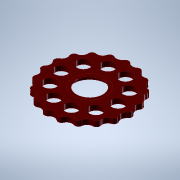
# Autodesk Inventor part: Rotor
Saved by Autodesk Inventor 2021 (Build 250183000, 183)
## iProperties
Created: 2022-08-28
Part Number: Rotor
Material: Ogólny
Document SubType Name: Modeling
Designer: MicnedSQ
Density: 1 g/cm^3
Appearance: Jasnoczerwona
Author: MicnedSQ
## iProperties of the stored document _Drukowanie 3D.ipt
Created: 2022-08-31
Part Number: _Drukowanie 3D
Material: Ogólny
Document SubType Name: Modeling
Designer: MicnedSQ
Density: 1 g/cm^3
Appearance: Domyślna
Author: MicnedSQ
Autodesk Inventor part; units mm, degrees
ref_plane "YZ Plane" through (0, 0, 0) normal (1, 0, 0) x (0, 1, 0)
ref_plane "XZ Plane" through (0, 0, 0) normal (0, 1, 0) x (-1, 0, 0)
ref_plane "XY Plane" through (0, 0, 0) normal (0, 0, 1) x (1, 0, 0)
sketch "Szkic1" plane through (0, 0, 0) normal (0, 1, 0) x (-1, 0, 0)
  spline S0 degree 5 poles (38.5, 0) (38.486, -0.9355) (38.7301, -1.8055) (39.0456, -2.7484) (39.8212, -3.5737) (40.5099, -4.4698) (40.6142, -4.6562) (40.8333, -5.1108) (40.9496, -5.6078) (40.9887, -5.8989) (41.0044, -6.5159) (40.8948, -7.12) (40.8044, -7.4298) (40.5885, -7.9454) (40.2744, -8.4095) (40.1203, -8.5919) (39.6992, -9.0108) (39.1783, -9.3014) (38.8791, -9.4777) (37.3997, -10.474) (36.3142, -11.9401) (35.8618, -13.4696) (36.0404, -15.1944) (36.6496, -16.773) (36.7512, -17.0218) (36.9128, -17.5238) (36.9474, -18.0505) (36.941, -18.3049) (36.8653, -18.8806) (36.6769, -19.4279) (36.5371, -19.7236) (36.2216, -20.2389) (35.8062, -20.6826) (35.5946, -20.8646) (35.1852, -21.1554) (34.728, -21.3438) (34.5206, -21.4137) (33.1558, -21.698) (31.793, -22.0921) (30.8042, -22.9138) (29.6475, -24.3964) (29.2399, -26.2198) (29.1454, -26.8625) (29.2627, -27.7313) (29.2011, -28.5914) (29.1537, -28.807) (29.0102, -29.3081) (28.7594, -29.7733) (28.5887, -30.0266) (28.1871, -30.5007) (27.6995, -30.8822) (27.4328, -31.0484) (26.9472, -31.2834) (26.426, -31.4138) (26.2028, -31.4498) (25.4759, -31.4825) (24.7564, -31.3259) (24.2597, -31.3096) (22.4191, -31.3724) (20.7296, -32.1668) (19.635, -33.1235) (18.9622, -34.5428) (18.5386, -36.0225) (18.4616, -36.2397) (18.2536, -36.6941) (17.9463, -37.0929) (17.7617, -37.2901) (17.31, -37.6816) (16.7902, -37.973) (16.4887, -38.1014) (15.923, -38.2724) (15.3331, -38.3261) (15.0679, -38.3226) (14.5636, -38.2676) (14.0874, -38.0997) (13.8701, -37.9997) (12.443, -37.2851) (10.8679, -36.8588) (9.3686, -37.0732) (7.6938, -37.8748) (6.4646, -39.2255) (6.191, -39.5691) (5.8381, -40.1537) (5.3451, -40.617) (5.1626, -40.7567) (4.6999, -41.0453) (4.1885, -41.2353) (3.8803, -41.3129) (3.269, -41.3994) (2.6488, -41.3603) (2.3525, -41.3079) (1.8482, -41.1691) (1.3948, -40.9271) (1.2077, -40.8149) (0.4846, -40.2055) (-0.1383, -39.4759) (-0.7752, -39.0861) (-2.4573, -38.2565) (-4.3399, -38.2442) (-5.5025, -38.4561) (-6.6123, -39.1858) (-7.6837, -39.9373) (-7.877, -40.0356) (-8.3311, -40.2356) (-8.8273, -40.3293) (-9.1094, -40.3566) (-9.7214, -40.3481) (-10.3147, -40.2173) (-10.6241, -40.1134) (-11.1431, -39.8723) (-11.6056, -39.5317) (-11.7893, -39.3635) (-12.1573, -38.9616) (-12.4116, -38.4794) (-12.5331, -38.216) (-13.3167, -36.6788) (-14.5397, -35.4012) (-16.0003, -34.7345) (-17.7967, -34.6208) (-19.4972, -35.064) (-19.7997, -35.1602) (-20.3453, -35.323) (-20.9136, -35.3357) (-21.1567, -35.3204) (-21.7162, -35.2238) (-22.2434, -35.0197) (-22.5316, -34.8691) (-23.0397, -34.5308) (-23.4728, -34.093) (-23.6512, -33.8673) (-23.9293, -33.4414) (-24.1006, -32.9737) (-24.1648, -32.7676) (-24.3431, -31.5633) (-24.4967, -30.3342) (-25.0291, -29.4057) (-26.199, -27.9263) (-27.907, -27.1334) (-28.7075, -26.8539) (-29.7585, -26.8736) (-30.7855, -26.7673) (-30.995, -26.7101) (-31.4778, -26.5536) (-31.9228, -26.2883) (-32.1623, -26.1137) (-32.6199, -25.6947) (-32.9801, -25.1958) (-33.1397, -24.9172) (-33.3591, -24.4108) (-33.4741, -23.8696) (-33.499, -23.6372) (-33.5086, -23.0043) (-33.3431, -22.3895) (-33.2706, -22.0056) (-33.0507, -20.2136) (-33.4922, -18.4251) (-34.3338, -17.1132) (-35.7229, -16.1585) (-37.2593, -15.5672) (-37.4951, -15.4755) (-37.9565, -15.2464) (-38.3521, -14.9145) (-38.5347, -14.7296) (-38.9012, -14.2715) (-39.1677, -13.7506) (-39.2841, -13.4443) (-39.4357, -12.8633) (-39.467, -12.2611) (-39.4522, -11.9868) (-39.3778, -11.4905) (-39.1962, -11.0287) (-39.0981, -10.8276) (-38.3366, -9.572) (-37.7222, -8.2083) (-37.7055, -6.8353) (-38.1425, -5.013) (-39.2807, -3.5467) (-39.6615, -3.1219) (-40.322, -2.6634) (-40.8495, -2.0714) (-40.9748, -1.8868) (-41.2394, -1.4286) (-41.4036, -0.9206) (-41.4684, -0.6174) (-41.5316, 0) (-41.4684, 0.6174) (-41.4036, 0.9206) (-41.2394, 1.4286) (-40.9748, 1.8868) (-40.8495, 2.0714) (-40.322, 2.6634) (-39.6615, 3.1219) (-39.2807, 3.5467) (-38.1425, 5.013) (-37.7055, 6.8353) (-37.7222, 8.2083) (-38.3366, 9.572) (-39.0981, 10.8276) (-39.1962, 11.0287) (-39.3778, 11.4905) (-39.4522, 11.9868) (-39.467, 12.2611) (-39.4357, 12.8633) (-39.2841, 13.4443) (-39.1677, 13.7506) (-38.9012, 14.2715) (-38.5347, 14.7296) (-38.3521, 14.9145) (-37.9565, 15.2464) (-37.4951, 15.4755) (-37.2593, 15.5672) (-35.7229, 16.1585) (-34.3338, 17.1132) (-33.4922, 18.4251) (-33.0507, 20.2136) (-33.2706, 22.0056) (-33.3431, 22.3895) (-33.5086, 23.0043) (-33.499, 23.6372) (-33.4741, 23.8696) (-33.3591, 24.4108) (-33.1397, 24.9172) (-32.9801, 25.1958) (-32.6199, 25.6947) (-32.1623, 26.1137) (-31.9228, 26.2883) (-31.4778, 26.5536) (-30.995, 26.7101) (-30.7855, 26.7673) (-29.7585, 26.8736) (-28.7075, 26.8539) (-27.907, 27.1334) (-26.199, 27.9263) (-25.0291, 29.4057) (-24.4967, 30.3342) (-24.3431, 31.5633) (-24.1648, 32.7676) (-24.1006, 32.9737) (-23.9293, 33.4414) (-23.6512, 33.8673) (-23.4728, 34.093) (-23.0397, 34.5308) (-22.5316, 34.8691) (-22.2434, 35.0197) (-21.7162, 35.2238) (-21.1567, 35.3204) (-20.9136, 35.3357) (-20.3453, 35.323) (-19.7997, 35.1602) (-19.4972, 35.064) (-17.7967, 34.6208) (-16.0003, 34.7345) (-14.5397, 35.4012) (-13.3167, 36.6788) (-12.5331, 38.216) (-12.4116, 38.4794) (-12.1573, 38.9616) (-11.7893, 39.3635) (-11.6056, 39.5317) (-11.1431, 39.8723) (-10.6241, 40.1134) (-10.3147, 40.2173) (-9.7214, 40.3481) (-9.1094, 40.3566) (-8.8273, 40.3293) (-8.3311, 40.2356) (-7.877, 40.0356) (-7.6837, 39.9373) (-6.6123, 39.1858) (-5.5025, 38.4561) (-4.3399, 38.2442) (-2.4573, 38.2565) (-0.7752, 39.0861) (-0.1383, 39.4759) (0.4846, 40.2055) (1.2077, 40.8149) (1.3948, 40.9271) (1.8482, 41.1691) (2.3525, 41.3079) (2.6488, 41.3603) (3.269, 41.3994) (3.8803, 41.3129) (4.1885, 41.2353) (4.6999, 41.0453) (5.1626, 40.7567) (5.3451, 40.617) (5.8381, 40.1537) (6.191, 39.5691) (6.4646, 39.2255) (7.6938, 37.8748) (9.3686, 37.0732) (10.8679, 36.8588) (12.443, 37.2851) (13.8701, 37.9997) (14.0874, 38.0997) (14.5636, 38.2676) (15.0679, 38.3226) (15.3331, 38.3261) (15.923, 38.2724) (16.4887, 38.1014) (16.7902, 37.973) (17.31, 37.6816) (17.7617, 37.2901) (17.9463, 37.0929) (18.2536, 36.6941) (18.4616, 36.2397) (18.5386, 36.0225) (18.9622, 34.5428) (19.635, 33.1235) (20.7296, 32.1668) (22.4191, 31.3724) (24.2597, 31.3096) (24.7564, 31.3259) (25.4759, 31.4825) (26.2028, 31.4498) (26.426, 31.4138) (26.9472, 31.2834) (27.4328, 31.0484) (27.6995, 30.8822) (28.1871, 30.5007) (28.5887, 30.0266) (28.7594, 29.7733) (29.0102, 29.3081) (29.1537, 28.807) (29.2011, 28.5914) (29.2627, 27.7313) (29.1454, 26.8625) (29.2399, 26.2198) (29.6475, 24.3964) (30.8042, 22.9138) (31.793, 22.0921) (33.1558, 21.698) (34.5206, 21.4137) (34.728, 21.3438) (35.1852, 21.1554) (35.5946, 20.8646) (35.8062, 20.6826) (36.2216, 20.2389) (36.5371, 19.7236) (36.6769, 19.4279) (36.8653, 18.8806) (36.941, 18.3049) (36.9474, 18.0505) (36.9128, 17.5238) (36.7512, 17.0218) (36.6496, 16.773) (36.0404, 15.1944) (35.8618, 13.4696) (36.3142, 11.9401) (37.3997, 10.474) (38.8791, 9.4777) (39.1783, 9.3014) (39.6992, 9.0108) (40.1203, 8.5919) (40.2744, 8.4095) (40.5885, 7.9454) (40.8044, 7.4298) (40.8948, 7.12) (41.0044, 6.5159) (40.9887, 5.8989) (40.9496, 5.6078) (40.8333, 5.1108) (40.6142, 4.6562) (40.5099, 4.4698) (39.8212, 3.5737) (39.0456, 2.7484) (38.7301, 1.8055) (38.486, 0.9355) (38.5, 0) knots 0 0 0 0 0 0 0.016204 0.016204 0.016204 0.019921 0.019921 0.019921 0.025097 0.025097 0.025097 0.030716 0.030716 0.030716 0.034915 0.034915 0.034915 0.04111 0.04111 0.04111 0.066147 0.066147 0.066147 0.070899 0.070899 0.070899 0.075375 0.075375 0.075375 0.081068 0.081068 0.081068 0.086001 0.086001 0.086001 0.089797 0.089797 0.089797 0.110671 0.110671 0.110671 0.122072 0.122072 0.122072 0.125893 0.125893 0.125893 0.131273 0.131273 0.131273 0.136766 0.136766 0.136766 0.140716 0.140716 0.140716 0.149555 0.149555 0.149555 0.172714 0.172714 0.172714 0.176745 0.176745 0.176745 0.1815 0.1815 0.1815 0.187212 0.187212 0.187212 0.191876 0.191876 0.191876 0.196074 0.196074 0.196074 0.220046 0.220046 0.220046 0.227884 0.227884 0.227884 0.231913 0.231913 0.231913 0.237453 0.237453 0.237453 0.242771 0.242771 0.242771 0.246539 0.246539 0.246539 0.259477 0.259477 0.259477 0.278884 0.278884 0.278884 0.282635 0.282635 0.282635 0.287652 0.287652 0.287652 0.293327 0.293327 0.293327 0.297709 0.297709 0.297709 0.302855 0.302855 0.302855 0.328039 0.328039 0.328039 0.333687 0.333687 0.333687 0.337977 0.337977 0.337977 0.343627 0.343627 0.343627 0.348727 0.348727 0.348727 0.352445 0.352445 0.352445 0.370293 0.370293 0.370293 0.384836 0.384836 0.384836 0.388573 0.388573 0.388573 0.393821 0.393821 0.393821 0.399406 0.399406 0.399406 0.403515 0.403515 0.403515 0.410488 0.410488 0.410488 0.435052 0.435052 0.435052 0.43951 0.43951 0.43951 0.444079 0.444079 0.444079 0.449786 0.449786 0.449786 0.454631 0.454631 0.454631 0.458528 0.458528 0.458528 0.480595 0.480595 0.480595 0.49068 0.49068 0.49068 0.49456 0.49456 0.49456 0.5 0.5 0.5 0.50544 0.50544 0.50544 0.50932 0.50932 0.50932 0.519405 0.519405 0.519405 0.541472 0.541472 0.541472 0.545369 0.545369 0.545369 0.550214 0.550214 0.550214 0.555921 0.555921 0.555921 0.56049 0.56049 0.56049 0.564948 0.564948 0.564948 0.589512 0.589512 0.589512 0.596485 0.596485 0.596485 0.600594 0.600594 0.600594 0.606179 0.606179 0.606179 0.611427 0.611427 0.611427 0.615164 0.615164 0.615164 0.629707 0.629707 0.629707 0.647555 0.647555 0.647555 0.651273 0.651273 0.651273 0.656373 0.656373 0.656373 0.662023 0.662023 0.662023 0.666313 0.666313 0.666313 0.671961 0.671961 0.671961 0.697145 0.697145 0.697145 0.702291 0.702291 0.702291 0.706673 0.706673 0.706673 0.712348 0.712348 0.712348 0.717365 0.717365 0.717365 0.721116 0.721116 0.721116 0.740523 0.740523 0.740523 0.753461 0.753461 0.753461 0.757229 0.757229 0.757229 0.762547 0.762547 0.762547 0.768087 0.768087 0.768087 0.772116 0.772116 0.772116 0.779954 0.779954 0.779954 0.803926 0.803926 0.803926 0.808124 0.808124 0.808124 0.812788 0.812788 0.812788 0.8185 0.8185 0.8185 0.823255 0.823255 0.823255 0.827286 0.827286 0.827286 0.850445 0.850445 0.850445 0.859284 0.859284 0.859284 0.863234 0.863234 0.863234 0.868727 0.868727 0.868727 0.874107 0.874107 0.874107 0.877928 0.877928 0.877928 0.889329 0.889329 0.889329 0.910203 0.910203 0.910203 0.913999 0.913999 0.913999 0.918932 0.918932 0.918932 0.924625 0.924625 0.924625 0.929101 0.929101 0.929101 0.933853 0.933853 0.933853 0.95889 0.95889 0.95889 0.965085 0.965085 0.965085 0.969284 0.969284 0.969284 0.974903 0.974903 0.974903 0.980079 0.980079 0.980079 0.983796 0.983796 0.983796 1 1 1 1 1 1
  circle A0 centre (-28, 0) radius 6.5
  circle A1 centre (0, 0) radius 16.05
  circle A2 centre (-22.6525, -16.458) radius 6.5
  circle A3 centre (-8.6525, -26.6296) radius 6.5
  circle A4 centre (8.6525, -26.6296) radius 6.5
  circle A5 centre (22.6525, -16.458) radius 6.5
  circle A6 centre (28, 0) radius 6.5
  circle A7 centre (22.6525, 16.458) radius 6.5
  circle A8 centre (8.6525, 26.6296) radius 6.5
  circle A9 centre (-8.6525, 26.6296) radius 6.5
  circle A10 centre (-22.6525, 16.458) radius 6.5
  dimension "d9" = 13
  dimension "d14" = 32.1
  dimension "d15" = 28
  dimension "d18" = 360
  constraints: 11 centre point, 1 coincident, 23 other
  measures "d9" diameter of A0
  measures "d14" diameter of A1
  measures "d15" distance of point (0, 0) A0.centre
extrude "Wyciągnięcie proste1" add sketch "Szkic1" along normal blind 5
sketch "Szkic2" plane through (0, 5, 0) normal (0, 1, 0) x (1, 0, 0)
  circle A0 centre (0, 0) radius 16
  circle A1 centre (0, 0) radius 13
  dimension "d23" = 32
  dimension "d24" = 26
  constraints: 2 centre point, 2 coincident
  measures "d23" diameter of A0
  measures "d24" diameter of A1
extrude "Wyciągnięcie proste2" add sketch "Szkic2" against normal blind 1
equation "curve S0 of \"Szkic1\": x = (45*cos(t))-(5*cos(t+atan(sin((1-20)*t)/((45/(1.5*20))-cos((1-20)*t)))))-(1.5*cos(20*t)); y = (-45*sin(t))+(5*sin(t+atan(sin((1-20)*t)/((45/(1.5*20))-cos((1-20)*t)))))+(1.5*s"
